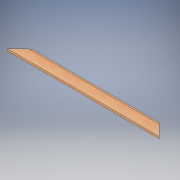
# Autodesk Inventor part: SkirtLength
Saved by Autodesk Inventor 2016 (Build 200138000, 138)
## iProperties
Created: 2016-02-11
Part Number: SkirtLength
Material: Wood (Birch)
Document SubType Name: Modeling
Designer: ron
Density: 0.55 g/cm^3
Appearance: Birch - Natural Polished
Mass: 1705.64 g
Surface Area: 4028.51 cm^2
Volume: 3101.17 cm^3
Author: ron
Autodesk Inventor part; units mm, degrees
ref_plane "YZ Plane" through (0, 0, 0) normal (1, 0, 0) x (0, 1, 0)
ref_plane "XZ Plane" through (0, 0, 0) normal (0, 1, 0) x (-1, 0, 0)
ref_plane "XY Plane" through (0, 0, 0) normal (0, 0, 1) x (1, 0, 0)
sketch "Sketch1" plane through (0, 0, 0) normal (1, 0, 0) x (0, 1, 0)
  line L0 (0, 0) -> (0, -127)
  line L1 (0, -127) -> (10, -127)
  line L2 (10, -127) -> (10, -101.6)
  line L3 (10, -101.6) -> (20, -101.6)
  line L4 (20, -101.6) -> (20, 0)
  line L5 (20, 0) -> (0, 0)
  dimension "d0" = 127
  dimension "d1" = 10
  dimension "d2" = 25.4
  dimension "d3" = 10
  constraints: 12 end point, 5 perpendicular, 1 vertical
  measures "d0" distance of L0.start L0.end
  measures "d1" distance of L0.end L1.end
  measures "d2" distance of L1.end L2.end
  measures "d3" distance of L2.end L3.end
extrude "Extrusion1" add sketch "Sketch1" along normal blind 1473.2
chamfer "Chamfer1" distance 127 angle 45 1 edges at (1473.2, 5, -127)
chamfer "Chamfer2" distance 127 angle 45 1 edges at (0, 5, -127)
sketch "Sketch2" plane through (0, 0, 0) normal (0, -1, 0) x (1, 0, 0)
  line L0 (101.6, -101.6) -> (1371.6, -101.6) projected
  line L1 (1346.2, -127) -> (1371.6, -101.6)
  line L2 (1473.2, 0) -> (1346.2, -127) projected
  line L3 (1371.6, -101.6) -> (1371.6, -76.2)
  line L4 (1371.6, -76.2) -> (1397, -76.2)
  line L5 (1371.6, -101.6) -> (1473.2, 0) projected
  point P0 (0, 0)
  dimension "d12" = 25.4
  constraints: 6 end point, 2 point on line, 1 collinear, 1 perpendicular, 1 vertical
  measures "d12" distance of L0.end L3.end
sketch "Sketch3" plane through (0, 0, 0) normal (0, -1, 0) x (1, 0, 0)
  line L0 (101.6, -101.6) -> (1371.6, -101.6) projected
  line L1 (101.6, -101.6) -> (101.6, -76.2)
  line L2 (101.6, -76.2) -> (76.2, -76.2)
  line L3 (0, 0) -> (101.6, -101.6) projected
  dimension "d13" = 25.4
  constraints: 4 end point, 1 perpendicular, 1 point on line, 1 vertical
  measures "d13" distance of L0.start L1.end
extrude "Extrusion2" cut sketch "Sketch2" against normal blind 3.175
extrude "Extrusion3" cut sketch "Sketch3" against normal blind 3.175
body "Solid1"
